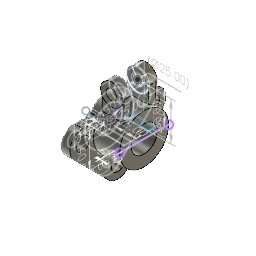
Erg2_7005 (Autodesk Fusion 360 design; units mm, degrees)
Autodesk Fusion 360 part; units mm, degrees
sketch "Sketch1" plane through (0, 0, 0) normal (1, 0, 0) x (0, 1, 0)
  circle A0 centre (0, 0) radius 15
  circle A1 centre (0, 0) radius 28
  circle A2 centre (0, -40) radius 7.5
  circle A3 centre (40, 0) radius 7.5
  circle A4 centre (-40, 0) radius 7.5
  arc A5 (-10.6066, -50.6066) -> (10.6066, -50.6066) centre (0, -40) ccw
  arc A6 (50.6066, -10.6066) -> (40, 15) centre (40, 0) ccw
  arc A7 (-40, 15) -> (-50.6066, -10.6066) centre (-40, 0) ccw
  line L0 (-50.6066, -10.6066) -> (-10.6066, -50.6066)
  line L1 (10.6066, -50.6066) -> (50.6066, -10.6066)
  line L2 (-40, 15) -> (-27.025, 15)
  line L3 (40, 15) -> (27.025, 15)
  arc A8 (-27.025, 15) -> (-22.025, 17.2887) centre (-26.7446, 20.9934) ccw
  arc A9 (22.025, 17.2887) -> (27.025, 15) centre (26.7446, 20.9934) ccw
  dimension "d1" = 30
  dimension "d2" = 56
  dimension "d3" = 15
  dimension "d4" = 40
  dimension "d5" = 15
  dimension "d6" = 15
  dimension "d8" = 80
  dimension "d9" = 40
  dimension "d10" = 15
  dimension "d11" = 15
  dimension "d12" = 15
  dimension "d13" = 6
  constraint coincident A0.centre A1.centre
  constraint concentric A0 A1
  constraint coincident A2.centre A5.centre
  constraint coincident A3.centre A6.centre
  constraint coincident A4.centre A7.centre
  constraint tangent A6 L1
  constraint tangent A5 L1
  constraint tangent A5 L0
  constraint tangent A7 L0
  constraint horizontal L2
  constraint tangent A7 L2
  constraint horizontal L3
  constraint tangent A6 L3
  constraint coincident A1 A8.end
  constraint tangent A1 A8
  constraint coincident A1 A9.start
  constraint tangent A1 A9
  measures "d1" diameter of A0
  measures "d2" diameter of A1
  measures "d3" diameter of A2
  measures "d4" distance of A0.centre A2.centre A1.centre
  measures "d5" diameter of A3
  measures "d6" diameter of A4
  measures "d8" distance of A3.centre A4.centre
  measures "d9" vertical distance of A2.centre A3.centre
  measures "d10" radius of A5
  measures "d11" radius of A6
  measures "d12" radius of A7
  measures "d13" radius of A8
extrude "Extrude1" add sketch "Sketch1" along normal blind 40 contours A1
extrude "Extrude2" add sketch "Sketch1" along normal blind 10 contours A1 A5 A6 A7 L0 L1 L2 L3 A8 A9
sketch "Sketch2" plane through (0, 0, 0) normal (0, 0, 1) x (1, 0, 0)
  line L0 (10, -18) -> (35, -18)
  line L1 (35, -18) -> (35, -10)
  line L2 (35, -10) -> (10, -10)
  line L3 (10, -10) -> (10, -18)
  line L4 (40, -28) -> (40, 28)
  line L5 (10, 10) -> (35, 10)
  line L6 (35, 10) -> (35, 18)
  line L7 (35, 18) -> (10, 18)
  line L8 (10, 18) -> (10, 10)
  dimension "d21" = 25
  dimension "d22" = 8
  dimension "d23" = 5
  dimension "d24" = 18
  constraint horizontal L0
  constraint vertical L1
  constraint horizontal L2
  constraint vertical L3
  constraint horizontal L5
  constraint vertical L6
  constraint horizontal L7
  constraint vertical L8
  measures "d21" distance of L1.end L2.end
  measures "d22" distance of L0.start L2.end
  measures "d23" distance of L0.end L4
  measures "d24" vertical distance of origin L0.end
extrude "Extrude3" add sketch "Sketch2" along normal blind 45 contours L0 L1 L2 L3
extrude "Extrude4" add sketch "Sketch2" along normal blind 45 contours L5 L6 L7 L8
delete_face "DeleteFace1" 1 faces at (26.6667, -10, 3.7268)
delete_face "DeleteFace2" 1 faces at (18.3333, 10, 7.4536)
delete_face "DeleteFace3" 1 faces at (35, -1.0568, 5.6199)
sketch "Sketch3" plane through (0, 10, 0) normal (0, -1, 0) x (1, 0, 0)
  line L0 (10, 26.1534) -> (35, 26.1534)
  line L1 (35, 26.1534) -> (35, 45)
  line L2 (35, 45) -> (10, 45)
  line L3 (10, 45) -> (10, 26.1534)
  circle A0 centre (22.5, 45) radius 12.5
  circle A1 centre (22.5, 45) radius 6
  dimension "d33" = 12
  dimension "d43" = 25
  dimension "d44" = 45
  constraint midpoint L2 A0.centre
  constraint coincident L1.end A0
  constraint concentric A0 A1
  measures "d33" diameter of A1
  measures "d43" diameter of A0
  measures "d44" vertical distance of A0.centre origin
extrude "Extrude5" add sketch "Sketch3" against normal blind 10 contours L2 A0 A1 | L2 A0 A1
extrude "Extrude6" cut sketch "Sketch3" against normal blind 10 contours L2 A1 picked at (24.5, 43.821)
sketch "Sketch4" plane through (0, -10, 0) normal (0, 1, 0) x (-1, 0, 0)
  line L0 (-35, 26.1534) -> (-10, 26.1534)
  line L1 (-10, 26.1534) -> (-10, 45)
  line L2 (-10, 45) -> (-35, 45)
  line L3 (-35, 45) -> (-35, 26.1534)
  circle A0 centre (-22.5, 45) radius 12.5
  circle A1 centre (-22.5, 45) radius 6
  dimension "d38" = 12
  constraint midpoint L2 A0.centre
  constraint coincident L1.end A0
  constraint concentric A0 A1
  measures "d38" diameter of A1
extrude "Extrude7" add sketch "Sketch4" against normal blind 10 contours L2 A0 A1 | L2 A0 A1
extrude "Extrude8" cut sketch "Sketch4" against normal blind 10 contours L2 A1 picked at (-20.5, 43.821)
